Autodesk Fusion 360 part; units mm, degrees
note: some values were not read from the file. Chosen so that the rebuilt part matches the saved one: which bodies a step acts on.
(part 2 of 2)
  line L292 (-102.87, -366.0775) -> (-102.87, -337.5025)
  line L293 (-102.87, -337.5025) -> (-74.295, -337.5025)
  line L294 (-74.295, -337.5025) -> (-74.295, -366.0775)
  line L295 (-74.295, -366.0775) -> (-102.87, -366.0775)
  line L296 (-136.2075, -366.0775) -> (-136.2075, -337.5025)
  line L297 (-136.2075, -337.5025) -> (-107.6325, -337.5025)
  line L298 (-107.6325, -337.5025) -> (-107.6325, -366.0775)
  line L299 (-107.6325, -366.0775) -> (-136.2075, -366.0775)
  line L300 (-169.545, -366.0775) -> (-169.545, -337.5025)
  line L301 (-169.545, -337.5025) -> (-140.97, -337.5025)
  line L302 (-140.97, -337.5025) -> (-140.97, -366.0775)
  line L303 (-140.97, -366.0775) -> (-169.545, -366.0775)
  line L304 (-202.8825, -366.0775) -> (-202.8825, -337.5025)
  line L305 (-202.8825, -337.5025) -> (-174.3075, -337.5025)
  line L306 (-174.3075, -337.5025) -> (-174.3075, -366.0775)
  line L307 (-174.3075, -366.0775) -> (-202.8825, -366.0775)
  line L308 (-236.22, -366.0775) -> (-236.22, -337.5025)
  line L309 (-236.22, -337.5025) -> (-207.645, -337.5025)
  line L310 (-207.645, -337.5025) -> (-207.645, -366.0775)
  line L311 (-207.645, -366.0775) -> (-236.22, -366.0775)
  line L312 (-269.5575, -366.0775) -> (-269.5575, -337.5025)
  line L313 (-269.5575, -337.5025) -> (-240.9825, -337.5025)
  line L314 (-240.9825, -337.5025) -> (-240.9825, -366.0775)
  line L315 (-240.9825, -366.0775) -> (-269.5575, -366.0775)
  line L316 (-302.895, -366.0775) -> (-302.895, -337.5025)
  line L317 (-302.895, -337.5025) -> (-274.32, -337.5025)
  line L318 (-274.32, -337.5025) -> (-274.32, -366.0775)
  line L319 (-274.32, -366.0775) -> (-302.895, -366.0775)
  line L320 (-336.2325, -366.0775) -> (-336.2325, -337.5025)
  line L321 (-336.2325, -337.5025) -> (-307.6575, -337.5025)
  line L322 (-307.6575, -337.5025) -> (-307.6575, -366.0775)
  line L323 (-307.6575, -366.0775) -> (-336.2325, -366.0775)
  line L324 (-369.57, -366.0775) -> (-369.57, -337.5025)
  line L325 (-369.57, -337.5025) -> (-340.995, -337.5025)
  line L326 (-340.995, -337.5025) -> (-340.995, -366.0775)
  line L327 (-340.995, -366.0775) -> (-369.57, -366.0775)
  line L328 (-69.5325, -399.415) -> (-69.5325, -370.84)
  line L329 (-69.5325, -370.84) -> (-40.9575, -370.84)
  line L330 (-40.9575, -370.84) -> (-40.9575, -399.415)
  line L331 (-40.9575, -399.415) -> (-69.5325, -399.415)
  line L332 (-369.57, -299.4025) -> (-369.57, -270.8275)
  line L333 (-369.57, -270.8275) -> (-340.995, -270.8275)
  line L334 (-340.995, -270.8275) -> (-340.995, -299.4025)
  line L335 (-340.995, -299.4025) -> (-369.57, -299.4025)
  line L336 (-336.2325, -299.4025) -> (-336.2325, -270.8275)
  line L337 (-336.2325, -270.8275) -> (-307.6575, -270.8275)
  line L338 (-307.6575, -270.8275) -> (-307.6575, -299.4025)
  line L339 (-307.6575, -299.4025) -> (-336.2325, -299.4025)
  line L340 (-302.895, -299.4025) -> (-302.895, -270.8275)
  line L341 (-302.895, -270.8275) -> (-274.32, -270.8275)
  line L342 (-274.32, -270.8275) -> (-274.32, -299.4025)
  line L343 (-274.32, -299.4025) -> (-302.895, -299.4025)
  line L344 (-269.5575, -299.4025) -> (-269.5575, -270.8275)
  line L345 (-269.5575, -270.8275) -> (-240.9825, -270.8275)
  line L346 (-240.9825, -270.8275) -> (-240.9825, -299.4025)
  line L347 (-240.9825, -299.4025) -> (-269.5575, -299.4025)
  line L348 (-236.22, -299.4025) -> (-236.22, -270.8275)
  line L349 (-236.22, -270.8275) -> (-207.645, -270.8275)
  line L350 (-207.645, -270.8275) -> (-207.645, -299.4025)
  line L351 (-207.645, -299.4025) -> (-236.22, -299.4025)
  line L352 (-202.8825, -299.4025) -> (-202.8825, -270.8275)
  line L353 (-202.8825, -270.8275) -> (-174.3075, -270.8275)
  line L354 (-174.3075, -270.8275) -> (-174.3075, -299.4025)
  line L355 (-174.3075, -299.4025) -> (-202.8825, -299.4025)
  line L356 (-169.545, -299.4025) -> (-169.545, -270.8275)
  line L357 (-169.545, -270.8275) -> (-140.97, -270.8275)
  line L358 (-140.97, -270.8275) -> (-140.97, -299.4025)
  line L359 (-140.97, -299.4025) -> (-169.545, -299.4025)
  line L360 (-136.2075, -299.4025) -> (-136.2075, -270.8275)
  line L361 (-136.2075, -270.8275) -> (-107.6325, -270.8275)
  line L362 (-107.6325, -270.8275) -> (-107.6325, -299.4025)
  line L363 (-107.6325, -299.4025) -> (-136.2075, -299.4025)
  line L364 (-102.87, -299.4025) -> (-102.87, -270.8275)
  line L365 (-102.87, -270.8275) -> (-74.295, -270.8275)
  line L366 (-74.295, -270.8275) -> (-74.295, -299.4025)
  line L367 (-74.295, -299.4025) -> (-102.87, -299.4025)
  line L368 (-69.5325, -299.4025) -> (-69.5325, -270.8275)
  line L369 (-69.5325, -270.8275) -> (-40.9575, -270.8275)
  line L370 (-40.9575, -270.8275) -> (-40.9575, -299.4025)
  line L371 (-40.9575, -299.4025) -> (-69.5325, -299.4025)
  line L372 (-369.57, -266.065) -> (-369.57, -237.49)
  line L373 (-369.57, -237.49) -> (-340.995, -237.49)
  line L374 (-340.995, -237.49) -> (-340.995, -266.065)
  line L375 (-340.995, -266.065) -> (-369.57, -266.065)
  line L376 (-336.2325, -266.065) -> (-336.2325, -237.49)
  line L377 (-336.2325, -237.49) -> (-307.6575, -237.49)
  line L378 (-307.6575, -237.49) -> (-307.6575, -266.065)
  line L379 (-307.6575, -266.065) -> (-336.2325, -266.065)
  line L380 (-302.895, -266.065) -> (-302.895, -237.49)
  line L381 (-302.895, -237.49) -> (-274.32, -237.49)
  line L382 (-274.32, -237.49) -> (-274.32, -266.065)
  line L383 (-274.32, -266.065) -> (-302.895, -266.065)
  line L384 (-269.5575, -266.065) -> (-269.5575, -237.49)
  line L385 (-269.5575, -237.49) -> (-240.9825, -237.49)
  line L386 (-240.9825, -237.49) -> (-240.9825, -266.065)
  line L387 (-240.9825, -266.065) -> (-269.5575, -266.065)
  line L388 (-236.22, -266.065) -> (-236.22, -237.49)
  line L389 (-236.22, -237.49) -> (-207.645, -237.49)
  line L390 (-207.645, -237.49) -> (-207.645, -266.065)
  line L391 (-207.645, -266.065) -> (-236.22, -266.065)
  line L392 (-202.8825, -266.065) -> (-202.8825, -237.49)
  line L393 (-202.8825, -237.49) -> (-174.3075, -237.49)
  line L394 (-174.3075, -237.49) -> (-174.3075, -266.065)
  line L395 (-174.3075, -266.065) -> (-202.8825, -266.065)
  line L396 (-169.545, -266.065) -> (-169.545, -237.49)
  line L397 (-169.545, -237.49) -> (-140.97, -237.49)
  line L398 (-140.97, -237.49) -> (-140.97, -266.065)
  line L399 (-140.97, -266.065) -> (-169.545, -266.065)
  line L400 (-136.2075, -266.065) -> (-136.2075, -237.49)
  line L401 (-136.2075, -237.49) -> (-107.6325, -237.49)
  line L402 (-107.6325, -237.49) -> (-107.6325, -266.065)
  line L403 (-107.6325, -266.065) -> (-136.2075, -266.065)
  line L404 (-102.87, -266.065) -> (-102.87, -237.49)
  line L405 (-102.87, -237.49) -> (-74.295, -237.49)
  line L406 (-74.295, -237.49) -> (-74.295, -266.065)
  line L407 (-74.295, -266.065) -> (-102.87, -266.065)
  line L408 (-69.5325, -266.065) -> (-69.5325, -237.49)
  line L409 (-69.5325, -237.49) -> (-40.9575, -237.49)
  line L410 (-40.9575, -237.49) -> (-40.9575, -266.065)
  line L411 (-40.9575, -266.065) -> (-69.5325, -266.065)
  line L412 (-36.195, -37.465) -> (-7.62, -37.465)
  line L413 (-7.62, -37.465) -> (-7.62, -66.04)
  line L414 (-7.62, -66.04) -> (-36.195, -66.04)
  line L415 (-36.195, -66.04) -> (-36.195, -37.465)
  line L416 (-402.9075, -66.04) -> (-402.9075, -37.465)
  line L417 (-402.9075, -37.465) -> (-374.3325, -37.465)
  line L418 (-374.3325, -37.465) -> (-374.3325, -66.04)
  line L419 (-374.3325, -66.04) -> (-402.9075, -66.04)
  line L420 (-69.5325, -99.3775) -> (-69.5325, -70.8025)
  line L421 (-69.5325, -70.8025) -> (-40.9575, -70.8025)
  line L422 (-40.9575, -70.8025) -> (-40.9575, -99.3775)
  line L423 (-40.9575, -99.3775) -> (-69.5325, -99.3775)
  line L424 (-102.87, -99.3775) -> (-102.87, -70.8025)
  line L425 (-102.87, -70.8025) -> (-74.295, -70.8025)
  line L426 (-74.295, -70.8025) -> (-74.295, -99.3775)
  line L427 (-74.295, -99.3775) -> (-102.87, -99.3775)
  line L428 (-136.2075, -99.3775) -> (-136.2075, -70.8025)
  line L429 (-136.2075, -70.8025) -> (-107.6325, -70.8025)
  line L430 (-107.6325, -70.8025) -> (-107.6325, -99.3775)
  line L431 (-107.6325, -99.3775) -> (-136.2075, -99.3775)
  line L432 (-169.545, -99.3775) -> (-169.545, -70.8025)
  line L433 (-169.545, -70.8025) -> (-140.97, -70.8025)
  line L434 (-140.97, -70.8025) -> (-140.97, -99.3775)
  line L435 (-140.97, -99.3775) -> (-169.545, -99.3775)
  line L436 (-202.8825, -99.3775) -> (-202.8825, -70.8025)
  line L437 (-202.8825, -70.8025) -> (-174.3075, -70.8025)
  line L438 (-174.3075, -70.8025) -> (-174.3075, -99.3775)
  line L439 (-174.3075, -99.3775) -> (-202.8825, -99.3775)
  line L440 (-236.22, -99.3775) -> (-236.22, -70.8025)
  line L441 (-236.22, -70.8025) -> (-207.645, -70.8025)
  line L442 (-207.645, -70.8025) -> (-207.645, -99.3775)
  line L443 (-207.645, -99.3775) -> (-236.22, -99.3775)
  line L444 (-269.5575, -99.3775) -> (-269.5575, -70.8025)
  line L445 (-269.5575, -70.8025) -> (-240.9825, -70.8025)
  line L446 (-240.9825, -70.8025) -> (-240.9825, -99.3775)
  line L447 (-240.9825, -99.3775) -> (-269.5575, -99.3775)
  line L448 (-302.895, -99.3775) -> (-302.895, -70.8025)
  line L449 (-302.895, -70.8025) -> (-274.32, -70.8025)
  line L450 (-274.32, -70.8025) -> (-274.32, -99.3775)
  line L451 (-274.32, -99.3775) -> (-302.895, -99.3775)
  line L452 (-336.2325, -99.3775) -> (-336.2325, -70.8025)
  line L453 (-336.2325, -70.8025) -> (-307.6575, -70.8025)
  line L454 (-307.6575, -70.8025) -> (-307.6575, -99.3775)
  line L455 (-307.6575, -99.3775) -> (-336.2325, -99.3775)
  line L456 (-369.57, -99.3775) -> (-369.57, -70.8025)
  line L457 (-369.57, -70.8025) -> (-340.995, -70.8025)
  line L458 (-340.995, -70.8025) -> (-340.995, -99.3775)
  line L459 (-340.995, -99.3775) -> (-369.57, -99.3775)
  line L460 (-69.5325, -132.715) -> (-69.5325, -104.14)
  line L461 (-69.5325, -104.14) -> (-40.9575, -104.14)
  line L462 (-40.9575, -104.14) -> (-40.9575, -132.715)
  line L463 (-40.9575, -132.715) -> (-69.5325, -132.715)
  line L464 (-102.87, -132.715) -> (-102.87, -104.14)
  line L465 (-102.87, -104.14) -> (-74.295, -104.14)
  line L466 (-74.295, -104.14) -> (-74.295, -132.715)
  line L467 (-74.295, -132.715) -> (-102.87, -132.715)
  line L468 (-136.2075, -132.715) -> (-136.2075, -104.14)
  line L469 (-136.2075, -104.14) -> (-107.6325, -104.14)
  line L470 (-107.6325, -104.14) -> (-107.6325, -132.715)
  line L471 (-107.6325, -132.715) -> (-136.2075, -132.715)
  line L472 (-169.545, -132.715) -> (-169.545, -104.14)
  line L473 (-169.545, -104.14) -> (-140.97, -104.14)
  line L474 (-140.97, -104.14) -> (-140.97, -132.715)
  line L475 (-140.97, -132.715) -> (-169.545, -132.715)
  line L476 (-202.8825, -132.715) -> (-202.8825, -104.14)
  line L477 (-202.8825, -104.14) -> (-174.3075, -104.14)
  line L478 (-174.3075, -104.14) -> (-174.3075, -132.715)
  line L479 (-174.3075, -132.715) -> (-202.8825, -132.715)
  line L480 (-236.22, -132.715) -> (-236.22, -104.14)
  line L481 (-236.22, -104.14) -> (-207.645, -104.14)
  line L482 (-207.645, -104.14) -> (-207.645, -132.715)
  line L483 (-207.645, -132.715) -> (-236.22, -132.715)
  line L484 (-269.5575, -132.715) -> (-269.5575, -104.14)
  line L485 (-269.5575, -104.14) -> (-240.9825, -104.14)
  line L486 (-240.9825, -104.14) -> (-240.9825, -132.715)
  line L487 (-240.9825, -132.715) -> (-269.5575, -132.715)
  line L488 (-7.62, -104.14) -> (-7.62, -132.715)
  line L489 (-7.62, -132.715) -> (-36.195, -132.715)
  line L490 (-36.195, -132.715) -> (-36.195, -104.14)
  line L491 (-36.195, -104.14) -> (-7.62, -104.14)
  line L492 (-36.195, -70.8025) -> (-7.62, -70.8025)
  line L493 (-7.62, -70.8025) -> (-7.62, -99.3775)
  line L494 (-7.62, -99.3775) -> (-36.195, -99.3775)
  line L495 (-36.195, -99.3775) -> (-36.195, -70.8025)
  line L496 (-374.3325, -399.415) -> (-402.9075, -399.415)
  line L497 (-402.9075, -399.415) -> (-402.9075, -370.84)
  line L498 (-402.9075, -370.84) -> (-374.3325, -370.84)
  line L499 (-374.3325, -370.84) -> (-374.3325, -399.415)
  line L500 (-374.3325, -337.5025) -> (-374.3325, -366.0775)
  line L501 (-374.3325, -366.0775) -> (-402.9075, -366.0775)
  line L502 (-402.9075, -366.0775) -> (-402.9075, -337.5025)
  line L503 (-402.9075, -337.5025) -> (-374.3325, -337.5025)
  line L504 (-374.3325, -304.165) -> (-374.3325, -332.74)
  line L505 (-374.3325, -332.74) -> (-402.9075, -332.74)
  line L506 (-402.9075, -332.74) -> (-402.9075, -304.165)
  line L507 (-402.9075, -304.165) -> (-374.3325, -304.165)
  line L508 (-374.3325, -270.8275) -> (-374.3325, -299.4025)
  line L509 (-374.3325, -299.4025) -> (-402.9075, -299.4025)
  line L510 (-402.9075, -299.4025) -> (-402.9075, -270.8275)
  line L511 (-402.9075, -270.8275) -> (-374.3325, -270.8275)
  line L512 (-374.3325, -237.49) -> (-374.3325, -266.065)
  line L513 (-374.3325, -266.065) -> (-402.9075, -266.065)
  line L514 (-402.9075, -266.065) -> (-402.9075, -237.49)
  line L515 (-402.9075, -237.49) -> (-374.3325, -237.49)
  line L516 (-374.3325, -204.1525) -> (-374.3325, -232.7275)
  line L517 (-374.3325, -232.7275) -> (-402.9075, -232.7275)
  line L518 (-402.9075, -232.7275) -> (-402.9075, -204.1525)
  line L519 (-402.9075, -204.1525) -> (-374.3325, -204.1525)
  line L520 (-374.3325, -170.815) -> (-374.3325, -199.39)
  line L521 (-374.3325, -199.39) -> (-402.9075, -199.39)
  line L522 (-402.9075, -199.39) -> (-402.9075, -170.815)
  line L523 (-402.9075, -170.815) -> (-374.3325, -170.815)
  line L524 (-374.3325, -137.4775) -> (-374.3325, -166.0525)
  line L525 (-374.3325, -166.0525) -> (-402.9075, -166.0525)
  line L526 (-402.9075, -166.0525) -> (-402.9075, -137.4775)
  line L527 (-402.9075, -137.4775) -> (-374.3325, -137.4775)
  line L528 (-374.3325, -104.14) -> (-374.3325, -132.715)
  line L529 (-374.3325, -132.715) -> (-402.9075, -132.715)
  line L530 (-402.9075, -132.715) -> (-402.9075, -104.14)
  line L531 (-402.9075, -104.14) -> (-374.3325, -104.14)
  line L532 (-402.9075, -70.8025) -> (-374.3325, -70.8025)
  line L533 (-374.3325, -70.8025) -> (-374.3325, -99.3775)
  line L534 (-374.3325, -99.3775) -> (-402.9075, -99.3775)
  line L535 (-402.9075, -99.3775) -> (-402.9075, -70.8025)
  line L536 (-40.9575, -37.465) -> (-40.9575, -66.04)
  line L537 (-40.9575, -66.04) -> (-69.5325, -66.04)
  line L538 (-69.5325, -66.04) -> (-69.5325, -37.465)
  line L539 (-69.5325, -37.465) -> (-40.9575, -37.465)
  line L540 (-102.87, -37.465) -> (-74.295, -37.465)
  line L541 (-74.295, -37.465) -> (-74.295, -66.04)
  line L542 (-74.295, -66.04) -> (-102.87, -66.04)
  line L543 (-102.87, -66.04) -> (-102.87, -37.465)
  line L544 (-369.57, -37.465) -> (-340.995, -37.465)
  line L545 (-340.995, -37.465) -> (-340.995, -66.04)
  line L546 (-340.995, -66.04) -> (-369.57, -66.04)
  line L547 (-369.57, -66.04) -> (-369.57, -37.465)
  line L548 (-336.2325, -37.465) -> (-307.6575, -37.465)
  line L549 (-307.6575, -37.465) -> (-307.6575, -66.04)
  line L550 (-307.6575, -66.04) -> (-336.2325, -66.04)
  line L551 (-336.2325, -66.04) -> (-336.2325, -37.465)
  line L552 (-302.895, -37.465) -> (-274.32, -37.465)
  line L553 (-274.32, -37.465) -> (-274.32, -66.04)
  line L554 (-274.32, -66.04) -> (-302.895, -66.04)
  line L555 (-302.895, -66.04) -> (-302.895, -37.465)
  line L556 (-269.5575, -37.465) -> (-240.9825, -37.465)
  line L557 (-240.9825, -37.465) -> (-240.9825, -66.04)
  line L558 (-240.9825, -66.04) -> (-269.5575, -66.04)
  line L559 (-269.5575, -66.04) -> (-269.5575, -37.465)
  line L560 (-236.22, -37.465) -> (-207.645, -37.465)
  line L561 (-207.645, -37.465) -> (-207.645, -66.04)
  line L562 (-207.645, -66.04) -> (-236.22, -66.04)
  line L563 (-236.22, -66.04) -> (-236.22, -37.465)
  line L564 (-202.8825, -37.465) -> (-174.3075, -37.465)
  line L565 (-174.3075, -37.465) -> (-174.3075, -66.04)
  line L566 (-174.3075, -66.04) -> (-202.8825, -66.04)
  line L567 (-202.8825, -66.04) -> (-202.8825, -37.465)
  line L568 (-169.545, -37.465) -> (-140.97, -37.465)
  line L569 (-140.97, -37.465) -> (-140.97, -66.04)
  line L570 (-140.97, -66.04) -> (-169.545, -66.04)
  line L571 (-169.545, -66.04) -> (-169.545, -37.465)
  line L572 (-136.2075, -37.465) -> (-107.6325, -37.465)
  line L573 (-107.6325, -37.465) -> (-107.6325, -66.04)
  line L574 (-107.6325, -66.04) -> (-136.2075, -66.04)
  line L575 (-136.2075, -66.04) -> (-136.2075, -37.465)
  line L576 (-407.67, -32.7025) -> (-407.67, -437.515)
  line L577 (-407.67, -437.515) -> (-2.8575, -437.515)
  line L578 (-2.8575, -437.515) -> (-2.8575, -32.7025)
  line L579 (-2.8575, -32.7025) -> (-407.67, -32.7025)
  line L580 (-136.2075, -432.7525) -> (-140.97, -432.7525)
  line L581 (-138.5888, -432.7525) -> (-138.5888, -437.515)
  line L582 (-269.5575, -432.7525) -> (-274.32, -432.7525)
  line L583 (-271.9388, -432.7525) -> (-271.9388, -437.515)
  line L584 (-7.62, -304.165) -> (-7.62, -299.4025)
  line L585 (-7.62, -301.7838) -> (-2.8575, -301.7838)
  line L586 (-7.62, -170.815) -> (-7.62, -166.0525)
  line L587 (-7.62, -168.4338) -> (-2.8575, -168.4338)
  line L588 (-138.5888, -437.515) -> (-138.8428, -437.515)
  line L589 (-138.8428, -437.515) -> (-138.8428, 19.685)
  line L590 (-138.8428, 19.685) -> (-138.5888, 19.685)
  line L591 (-138.5888, 19.685) -> (-138.5888, -437.515)
  line L592 (-271.9388, -437.515) -> (-271.6848, -437.515)
  line L593 (-271.6848, -437.515) -> (-271.6848, 19.685)
  line L594 (-271.6848, 19.685) -> (-271.9388, 19.685)
  line L595 (-271.9388, 19.685) -> (-271.9388, -437.515)
  line L596 (-2.8575, -301.7838) -> (-460.0575, -301.7838)
  line L597 (-460.0575, -301.7838) -> (-460.0575, -302.0378)
  line L598 (-460.0575, -302.0378) -> (-2.8575, -302.0378)
  line L599 (-2.8575, -302.0378) -> (-2.8575, -301.7838)
  line L600 (-2.8575, -168.4338) -> (-460.0575, -168.4338)
  line L601 (-460.0575, -168.4338) -> (-460.0575, -168.6878)
  line L602 (-460.0575, -168.6878) -> (-2.8575, -168.6878)
  line L603 (-2.8575, -168.6878) -> (-2.8575, -168.4338)
  dimension "d13" = 457.2
  dimension "d14" = 0.254
  dimension "d15" = 0.254
  dimension "d16" = 457.2
  dimension "d17" = 0.254
  dimension "d18" = 457.2
  dimension "d19" = 457.2
  dimension "d20" = 0.254
  constraint coincident L144.end L145.start
  constraint coincident L140.start L143.end
  constraint midpoint L580 L581.start
  constraint coincident L577 L581.end
  constraint perpendicular L577 L581
  constraint coincident L216.end L217.start
  constraint coincident L212.start L215.end
  constraint midpoint L582 L583.start
  constraint coincident L577 L583.end
  constraint perpendicular L577 L583
  constraint coincident L220.start L223.end
  constraint coincident L228.end L229.start
  constraint midpoint L584 L585.start
  constraint coincident L578 L585.end
  constraint perpendicular L578 L585
  constraint coincident L240.start L243.end
  constraint coincident L244.end L245.start
  constraint midpoint L586 L587.start
  constraint coincident L578 L587.end
  constraint perpendicular L578 L587
  constraint horizontal L588
  constraint vertical L589
  constraint horizontal L590
  constraint vertical L591
  constraint horizontal L592
  constraint vertical L593
  constraint horizontal L594
  constraint vertical L595
  constraint horizontal L596
  constraint vertical L597
  constraint horizontal L598
  constraint vertical L599
  constraint horizontal L600
  constraint vertical L601
  constraint horizontal L602
  constraint vertical L603
  measures "d13" distance of L581.end L590.end
  measures "d14" distance of L581.end L588.end
  measures "d15" distance of L583.end L592.end
  measures "d16" distance of L583.end L594.end
  measures "d17" distance of L585.end L598.end
  measures "d18" distance of L585.end L596.end
  measures "d19" distance of L587.end L600.end
  measures "d20" distance of L587.end L602.end
extrude "Extrude2" cut sketch "Sketch2" against normal blind 38.1 contours L576 L595 L600 L602 | L579 L593 L595 L600 | L593 L595 L600 L602 | L576 L595 L596 L598 | L593 L595 L596 L602 | L589 L593 L600 L602 | L579 L589 L591 L600 | L589 L591 L600 L602 | L582 L593 L595 L598 | L589 L593 L596 L598 | L589 L591 L596 L602 | L586 L591 L600 L602 | L577 L582 L583 L592 L593 L595 | L589 L591 L596 L598 | L578 L586 L587 L600 L602 L603 | L580 L589 L591 L598 | L584 L591 L596 L598 | L577 L580 L581 L588 L589 L591 | L578 L584 L585 L596 L598 L599 bodies 1 makes body 4 at (60.8013, 435.9275, 0) makes body 6 at (194.945, 435.9275, 0) makes body 6 at (271.8541, 302.0378, 6.35) makes body 6 at (406.0825, 245.5122, 0) makes body 2 at (340.2013, 34.29, 0) makes body 3 at (204.47, 34.29, 19.05) makes body 5 at (70.3263, 34.29, 0) makes body 6 at (150.495, 235.9025, 0) makes body 6 at (406.0825, 379.6559, 0)
extrude "Extrude3" cut 1 faces at (271.7694, 301.9531, 19.05) along direction (0, 0, -1) blind 45.72 on bodies 6 bodies 6 makes body 7 at (406.0825, 245.5122, 0) makes body 8 at (150.495, 235.9025, 0) makes body 9 at (194.945, 435.9275, 0)
equation "d5 = 1.125 in + 0.1875 in"
equation "d6 = 1.125 in + 0.1875 in"
